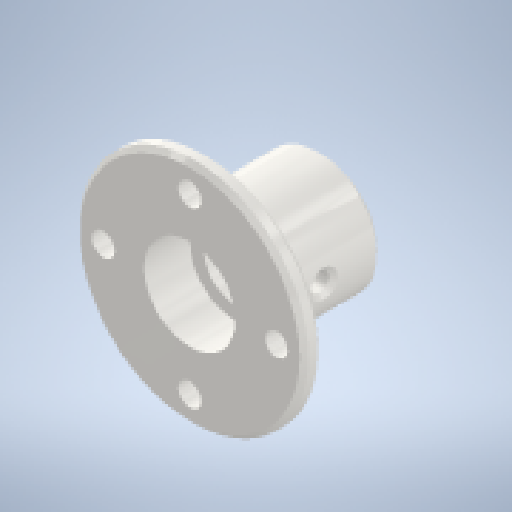
# Autodesk Inventor part: 22 - Valve Disc Hub
Saved by Autodesk Inventor 2025.2 (Build 292293000, 293)
## iProperties
Created: 2025-07-17
Part Number: 22 - Valve Disc Hub
Material: Steel AISI 1020 108 ANLD
Document SubType Name: Modeling
Designer: bless
Density: 7.87 g/cm^3
Appearance: Steel
Author: bless
Autodesk Inventor part; units mm, degrees
ref_plane "YZ Plane" through (0, 0, 0) normal (1, 0, 0) x (0, 1, 0)
ref_plane "XZ Plane" through (0, 0, 0) normal (0, 1, 0) x (-1, 0, 0)
ref_plane "XY Plane" through (0, 0, 0) normal (0, 0, 1) x (1, 0, 0)
sketch "Sketch1" plane through (0, 0, 0) normal (0, 0, 1) x (1, 0, 0)
  circle A0 centre (0, 0) radius 12.5
  dimension "d0" = 25
  constraints: 1 centre point, 1 coincident
  measures "d0" diameter of A0
extrude "Extrusion1" add sketch "Sketch1" along normal blind 2
sketch "Sketch2" plane through (0, 0, 0) normal (0, 0, -1) x (-1, 0, 0)
  circle A0 centre (0, 0) radius 12.5 projected
  circle A1 centre (0, 0) radius 6.5
  dimension "d3" = 13
  constraints: 1 centre point, 1 coincident
  measures "d3" diameter of A1
extrude "Extrusion2" add sketch "Sketch2" along normal blind 12.5 contours A1
sketch "Sketch3" plane through (0, 0, 2) normal (0, 0, 1) x (1, 0, 0)
  circle A0 centre (0, 0) radius 12.5 projected
  circle A1 centre (0, 0) radius 5
  dimension "d6" = 10
  constraints: 1 centre point, 1 coincident
  measures "d6" diameter of A1
extrude "Extrusion3" cut sketch "Sketch3" against normal blind 5 contours A1
sketch "Sketch4" plane through (0, 0, -3) normal (0, 0, 1) x (1, 0, 0)
  circle A0 centre (0, 0) radius 5 projected
  circle A1 centre (0, 0) radius 3.5
  dimension "d9" = 7
  constraints: 1 centre point, 1 coincident
  measures "d9" diameter of A1
extrude "Extrusion4" cut sketch "Sketch4" against normal blind 8 contours A1
sketch "Sketch5" plane through (0, 0, -11) normal (0, 0, 1) x (1, 0, 0)
  circle A0 centre (0, 0) radius 3.5 projected
  circle A1 centre (0, 0) radius 2.5
  dimension "d12" = 5
  constraints: 1 centre point, 1 coincident
  measures "d12" diameter of A1
extrude "Extrusion5" cut sketch "Sketch5" against normal through all contours A1
sketch "Sketch6" plane through (0, 0, 0) normal (1, 0, 0) x (0, 1, 0)
  line L0 (-6.5, -12.5) -> (6.5, -12.5) projected
  line L1 (6.5, 0) -> (-6.5, 0) projected
  line L2 (6.5, 0) -> (6.5, -12.5) projected
  line L3 (-6.5, 0) -> (-6.5, -12.5) projected
  point P0 (0, 0)
  point P1 (0, -6.25)
hole "Hole1" at (0, 0, -6.25) direction (1, 0, 0) diameter 2 end through all
chamfer "Chamfer1" distance 0.5 angle 45 4 edges at (-12.5, 0, 2) (-12.5, 0, 0) (6.5, 0, -12.5) (6.5, 0.0019, -7.25)
sketch "Sketch7" plane through (0, 0, 2) normal (0, 0, 1) x (1, 0, 0)
  circle A0 centre (0, 0) radius 12 projected
  circle A1 centre (0, 0) radius 9.5
  circle A2 centre (0, 0) radius 3.5 construction
  line L0 (0, 0) -> (12, 0) construction
  circle A3 centre (0, 0) radius 2.5 construction
  line L1 (0, 0) -> (6.7175, 6.7175) construction
  circle A4 centre (6.7175, 6.7175) radius 1.25
  circle A5 centre (6.7175, -6.7175) radius 1.25
  circle A6 centre (-6.7175, -6.7175) radius 1.25
  circle A7 centre (-6.7175, 6.7175) radius 1.25
  point P0 (0, 9.5)
  point P1 (0, -9.5)
  point P2 (-9.5, 0)
  point P3 (9.5, 0)
  dimension "d25" = 19
  dimension "d26" = 45
  dimension "d29" = 360
  dimension "d31" = 2.5
  dimension "d32" = 2.5
  dimension "d33" = 2.5
  dimension "d34" = 2.5
  constraints: 5 centre point, 5 coincident, 5 point on circle, 4 end point, 1 horizontal, 1 horizontal alignment, 6 other
  measures "d25" diameter of A1
  measures "d26" angle of L0 L1
  measures "d31" diameter of A4
  measures "d32" diameter of A5
  measures "d33" diameter of A6
  measures "d34" diameter of A7
extrude "Extrusion6" cut sketch "Sketch7" against normal through all contours A4 A1 | A1 A4 | A5 A1 | A1 A5 | A7 A1 | A1 A7 | A6 A1 | A1 A6
body "Solid1"
